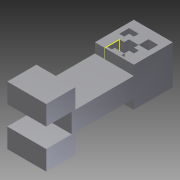
# Autodesk Inventor part: Creeper
Saved by Autodesk Inventor 2012 (Build 160160000, 160)
## iProperties
Created: 2011-09-15
Part Number: Creeper
Document SubType Name: Modeling
Designer: 09gavalchink
Density: 1 g/cm^3
Material: Default
Author: 09gavalchink
Autodesk Inventor part; units mm, degrees
ref_plane "YZ Plane" through (0, 0, 0) normal (1, 0, 0) x (0, 1, 0)
ref_plane "XZ Plane" through (0, 0, 0) normal (0, 1, 0) x (-1, 0, 0)
ref_plane "XY Plane" through (0, 0, 0) normal (0, 0, 1) x (1, 0, 0)
sketch "Sketch1" plane through (0, 0, 0) normal (0, 0, 1) x (1, 0, 0)
  line L0 (-101.6, 50.8) -> (0, 50.8)
  line L1 (0, 50.8) -> (0, 0)
  line L2 (0, 0) -> (-101.6, 0)
  line L3 (-101.6, 0) -> (-101.6, 50.8)
  dimension "d0" = 101.6
  dimension "d1" = 50.8
  constraints: 8 end point, 2 parallel, 1 horizontal, 1 perpendicular
  measures "d0" distance of L0.start L0.end
  measures "d1" distance of L2.end L0.start
extrude "Extrusion1" add sketch "Sketch1" along normal blind 76.2
sketch "Sketch2" plane through (-101.6, 0, 0) normal (0, -1, 0) x (1, 0, 0)
  line L0 (0, 0) -> (0, 76.2) projected
  line L1 (101.6, 0) -> (0, 0)
  line L2 (0, 0) -> (0, 9.5563)
  line L3 (0, 9.5563) -> (101.6, 9.5563)
  line L4 (101.6, 9.5563) -> (101.6, 0)
  constraints: 8 end point, 2 parallel, 1 horizontal, 1 perpendicular, 1 point on line
extrude "Extrusion2" add sketch "Sketch2" along normal blind 50.8
sketch "Sketch3" plane through (0, 0, 0) normal (0, 0, -1) x (-1, 0, 0)
  line L0 (101.6, -50.8) -> (0, -50.8)
  line L1 (0, -50.8) -> (0, -101.6194)
  line L2 (0, -101.6194) -> (101.6, -101.6194)
  line L3 (101.6, -101.6194) -> (101.6, -50.8)
  point P0 (0, 0)
  constraints: 8 end point, 2 parallel, 1 horizontal, 1 perpendicular
extrude "Extrusion3" add sketch "Sketch3" against normal blind 76.2
sketch "Sketch4" plane through (0, 0, 0) normal (0, 0, -1) x (-1, 0, 0)
  line L0 (0, -101.6194) -> (0, 50.8) projected
  line L1 (101.6, 50.8) -> (101.6, -101.6194) projected
  line L2 (101.6, 0) -> (0, 0)
  line L3 (0, 0) -> (0, -50.8671)
  line L4 (0, -50.8671) -> (101.6, -50.8671)
  line L5 (101.6, -50.8671) -> (101.6, 0)
  point P0 (0, 0)
  constraints: 8 end point, 2 parallel, 2 point on line, 1 horizontal, 1 perpendicular
extrude "Extrusion4" add sketch "Sketch4" along normal blind 152.4
sketch "Sketch5" plane through (0, 0, -152.4) normal (0, 0, -1) x (-1, 0, 0)
  line L0 (0, -76.278) -> (101.6, -76.278)
  line L1 (101.6, -76.278) -> (101.6, 25.322)
  line L2 (101.6, 25.322) -> (0, 25.322)
  line L3 (0, 25.322) -> (0, -76.278)
  dimension "d10" = 101.6
  dimension "d11" = 101.6
  constraints: 8 end point, 2 parallel, 1 horizontal, 1 perpendicular
  measures "d10" distance of L2.end L0.start
  measures "d11" distance of L0.start L0.end
extrude "Extrusion5" add sketch "Sketch5" along normal blind 101.6
sketch "Sketch6" plane through (-101.6, 25.322, -152.4) normal (0, 1, 0) x (1, 0, 0)
  line L0 (0, 0) -> (101.6, 0) projected
  line L1 (12.7038, 76.4129) -> (38.1038, 76.4129)
  line L2 (38.1038, 76.4129) -> (38.1038, 51.0129)
  line L3 (38.1038, 51.0129) -> (12.7038, 51.0129)
  line L4 (12.7038, 51.0129) -> (12.7038, 76.4129)
  line L5 (63.1592, 76.7092) -> (88.5592, 76.7092)
  line L6 (88.5592, 76.7092) -> (88.5592, 51.3092)
  line L7 (88.5592, 51.3092) -> (63.1592, 51.3092)
  line L8 (63.1592, 51.3092) -> (63.1592, 76.7092)
  line L9 (37.1295, 0) -> (29.2048, 0)
  point P0 (101.6, -152.4)
  dimension "d14" = 25.4
  dimension "d15" = 25.4
  dimension "d16" = 25.4
  dimension "d17" = 25.4
  constraints: 18 end point, 4 parallel, 3 horizontal, 2 perpendicular, 1 point on line
  measures "d14" distance of L1.start L1.end
  measures "d15" distance of L3.end L1.start
  measures "d16" distance of L5.end L6.end
  measures "d17" distance of L5.start L5.end
extrude "Extrusion6" cut sketch "Sketch6" against normal blind 25.4
sketch "Sketch7" plane through (-101.6, 25.322, -152.4) normal (0, 1, 0) x (1, 0, 0)
  line L0 (25.3513, 38.6799) -> (38.4727, 38.6799)
  line L1 (38.4727, 38.6799) -> (38.4727, 0.5799)
  line L2 (38.4727, 0.5799) -> (25.3513, 0.5799)
  line L3 (25.3513, 0.5799) -> (25.3513, 38.6799)
  line L4 (64.117, 38.5479) -> (76.0531, 38.5479)
  line L5 (76.0531, 38.5479) -> (76.0531, 0.4479)
  line L6 (76.0531, 0.4479) -> (64.117, 0.4479)
  line L7 (64.117, 0.4479) -> (64.117, 38.5479)
  point P0 (101.6, -152.4)
  dimension "d20" = 38.1
  dimension "d21" = 38.1
  constraints: 16 end point, 4 parallel, 2 horizontal, 2 perpendicular
  measures "d20" distance of L2.end L0.start
  measures "d21" distance of L4.end L5.end
extrude "Extrusion7" cut sketch "Sketch7" against normal blind 25.4
sketch "Sketch8" plane through (-101.6, 25.322, -152.4) normal (0, 1, 0) x (1, 0, 0)
  line L0 (76.0531, 38.5479) -> (76.0531, 0.4479) projected
  line L1 (25.3513, 38.6799) -> (76.0531, 38.6799)
  line L2 (76.0531, 38.6799) -> (76.0531, 13.2799)
  line L3 (76.0531, 13.2799) -> (25.3513, 13.2799)
  line L4 (25.3513, 13.2799) -> (25.3513, 38.6799)
  point P0 (101.6, -152.4)
  dimension "d24" = 25.4
  constraints: 8 end point, 2 parallel, 1 horizontal, 1 perpendicular, 1 point on line
  measures "d24" distance of L3.end L1.start
extrude "Extrusion8" cut sketch "Sketch8" against normal blind 25.4
sketch "Sketch9" plane through (-76.2487, 25.322, -152.9799) normal (1, 0, 0) x (0, 0, -1)
  line L0 (0, 0) -> (38.1, 0) projected
  line L1 (0, 0) -> (0, -25.4) projected
  line L2 (38.1, -25.4) -> (0, -25.4) projected
  line L3 (38.1, 0) -> (38.1, -25.4) projected
  point P0 (-152.9799, -25.322)
sketch "Sketch10" plane through (-101.6, 25.322, -152.4) normal (0, 1, 0) x (1, 0, 0)
  line L0 (25.3513, 38.6799) -> (76.0531, 38.6799) projected
  line L1 (38.1038, 51.0129) -> (63.1592, 51.0129)
  line L2 (63.1592, 51.0129) -> (63.1592, 38.6799)
  line L3 (63.1592, 38.6799) -> (38.1038, 38.6799)
  line L4 (38.1038, 38.6799) -> (38.1038, 51.0129)
  point P0 (101.6, -152.4)
  constraints: 8 end point, 2 parallel, 1 horizontal, 1 perpendicular, 1 point on line
extrude "Extrusion9" cut sketch "Sketch10" against normal blind 25.4
sketch "Sketch11" plane through (-101.6, -0.078, -152.4) normal (0, 1, 0) x (1, 0, 0)
  line L0 (88.5592, 76.7092) -> (75.8592, 76.7092)
  line L1 (75.8592, 76.7092) -> (75.8592, 64.0092)
  line L2 (75.8592, 64.0092) -> (88.5592, 64.0092)
  line L3 (88.5592, 64.0092) -> (88.5592, 76.7092)
  point P0 (101.6, -152.4)
  constraints: 8 end point, 2 parallel, 1 horizontal, 1 perpendicular
extrude "Extrusion10" add sketch "Sketch11" along normal blind 12.7
sketch "Sketch12" plane through (-101.6, -0.078, -152.4) normal (0, 1, 0) x (1, 0, 0)
  line L0 (12.7038, 76.4129) -> (25.4038, 76.4129)
  line L1 (25.4038, 76.4129) -> (25.4038, 63.4415)
  line L2 (25.4038, 63.4415) -> (12.7038, 63.4415)
  line L3 (12.7038, 63.4415) -> (12.7038, 76.4129)
  point P0 (101.6, -152.4)
  constraints: 8 end point, 2 parallel, 1 horizontal, 1 perpendicular
extrude "Extrusion11" add sketch "Sketch12" along normal blind 12.7
sketch "Sketch13" plane through (-63.1273, 25.322, -152.9799) normal (0, 0, -1) x (-1, 0, 0)
  line L0 (13.1215, -25.4) -> (0, -25.4) projected
  line L1 (13.1215, 0) -> (13.1215, -25.4) projected
  line L2 (0, 0) -> (13.1215, 0) projected
  line L3 (0, 0) -> (0, -25.4) projected
  point P0 (-63.1273, -25.322)
extrude "Extrusion12" add sketch "Sketch13" along normal blind 5.08
sketch "Sketch14" plane through (-25.5469, 25.322, -152.8479) normal (0, 0, -1) x (-1, 0, 0)
  line L0 (11.9361, -25.4) -> (0, -25.4) projected
  line L1 (11.9361, 0) -> (11.9361, -25.4) projected
  line L2 (0, 0) -> (11.9361, 0) projected
  line L3 (0, 0) -> (0, -25.4) projected
  point P0 (-25.5469, -25.322)
extrude "Extrusion13" add sketch "Sketch14" along normal blind 5.08
body "Solid1"
